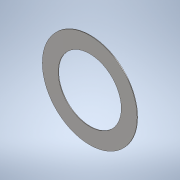
# Autodesk Inventor part: ChainTensionerBearingShim
Saved by Autodesk Inventor 2022 (Build 260153000, 153)
## iProperties
Created: 2021-06-19
Part Number: ChainTensionerBearingShim
Material: Stainless Steel, 440C
Catalog Web Link: https://www.mcmaster.com/97022A333/
Document SubType Name: Modeling
Designer: M3rob
Density: 7.75 g/cm^3
Appearance: Semi-Polished
Title: 97022A333
Author: Matthew Lydon
Autodesk Inventor part; units mm, degrees
ref_plane "YZ Plane" through (0, 0, 0) normal (1, 0, 0) x (0, 1, 0)
ref_plane "XZ Plane" through (0, 0, 0) normal (0, 1, 0) x (-1, 0, 0)
ref_plane "XY Plane" through (0, 0, 0) normal (0, 0, 1) x (1, 0, 0)
sketch "Sketch1" plane through (0, 0, 0) normal (0, 0, 1) x (1, 0, 0)
  circle A0 centre (0, 0) radius 6.35
  circle A1 centre (0, 0) radius 9.525
  dimension "d0" = 12.7
  dimension "d1" = 19.05
  constraints: 2 centre point, 2 coincident
  measures "d0" diameter of A0
  measures "d1" diameter of A1
extrude "Extrusion1" add sketch "Sketch1" along normal mid plane 0.127
body "Solid1"
